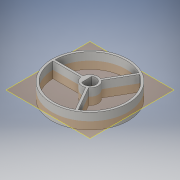
# Autodesk Inventor part: Wheel
Saved by Autodesk Inventor 2016 (Build 200138000, 138)
## iProperties
Created: 2016-02-09
Part Number: Wheel
Material: Generic
Document SubType Name: Modeling
Designer: Michael
Density: 1 g/cm^3
Appearance: Default
Author: Michael
Autodesk Inventor part; units mm, degrees
ref_plane "YZ Plane" through (0, 0, 0) normal (1, 0, 0) x (0, 1, 0)
ref_plane "XZ Plane" through (0, 0, 0) normal (0, 1, 0) x (-1, 0, 0)
ref_plane "XY Plane" through (0, 0, 0) normal (0, 0, 1) x (1, 0, 0)
sketch "Sketch1" plane through (0, 0, 0) normal (0, 1, 0) x (-1, 0, 0)
  circle A0 centre (0, 0) radius 25
  circle A1 centre (0, 0) radius 3.95
  line L0 (2.1, -3.3455) -> (2.1, 3.3455)
  dimension "d2" = 50
  dimension "d3" = 7.9
  dimension "d4" = 2.1
  constraints: 2 centre point, 2 coincident, 2 end point, 2 point on circle, 1 vertical
  measures "d2" diameter of A0
  measures "d3" diameter of A1
  measures "d4" distance from line of point (0, 0) L0
extrude "Extrusion1" add sketch "Sketch1" along normal blind 10 contours A0 | A1 L0 picked at (2.7167, 0)
ref_plane "Work Plane1" through (0, 5, 0) normal (0, 1, 0) x (1, 0, 0)
sketch "Sketch2" plane through (0, 10, 0) normal (0, 1, 0) x (1, 0, 0)
  arc A0 (-2.1, -3.3455) -> (-2.1, 3.3455) centre (0, 0) ccw projected
  line L0 (-2.1, -3.3455) -> (-2.1, 3.3455) projected
  circle A1 centre (0, 0) radius 25 projected
  circle A2 centre (0, 0) radius 25 projected
  line L1 (-23.5896, -0.7) -> (-5.304, -0.7)
  line L2 (-23.5896, 0.7) -> (-5.304, 0.7)
  line L3 (12.401, 20.0792) -> (3.2582, 4.2434)
  line L4 (11.1886, 20.7792) -> (2.0458, 4.9434)
  line L5 (11.1886, -20.7792) -> (2.0458, -4.9434)
  line L6 (12.401, -20.0792) -> (3.2582, -4.2434)
  arc A3 (2.0458, 4.9434) -> (-5.304, 0.7) centre (0, 0) ccw
  arc A4 (-5.304, -0.7) -> (2.0458, -4.9434) centre (0, 0) ccw
  arc A5 (3.2582, -4.2434) -> (3.2582, 4.2434) centre (0, 0) ccw
  arc A6 (11.1886, 20.7792) -> (-23.5896, 0.7) centre (0, 0) ccw
  arc A7 (-23.5896, -0.7) -> (11.1886, -20.7792) centre (0, 0) ccw
  arc A8 (12.401, -20.0792) -> (12.401, 20.0792) centre (0, 0) ccw
  dimension "d9" = 1.4
  dimension "d12" = 360
  constraints: 12 end point, 12 point on circle, 6 centre point, 3 coincident, 2 parallel, 1 horizontal, 20 other
  measures "d9" distance between parallel lines of L2 L1
extrude "Extrusion2" cut sketch "Sketch2" against normal blind 10 contours L1 A4 L5 A7 | A6 L4 A3 L2 | A8 L6 A5 L3
body "Solid1"
